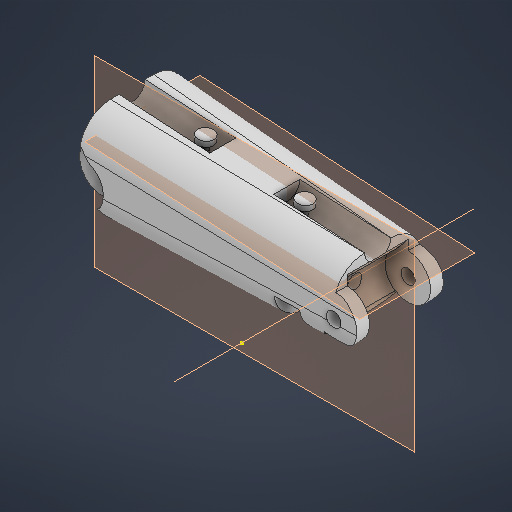
# Autodesk Inventor part: falange1_inidice_V13
Saved by Autodesk Inventor 2026.1 (Build 301233020, 233B)
## iProperties
Created: 2026-01-14
Part Number: falange1_inidice_V13
Material: Generic
Document SubType Name: Modeling
Designer: user
Density: 1 g/cm^3
Appearance: Default
Author: user
Autodesk Inventor part; units mm, degrees
ref_plane "YZ Plane" through (0, 0, 0) normal (1, 0, 0) x (0, 1, 0)
sketch "Sketch1" plane through (0, 0, 0) normal (0, 0, 1) x (1, 0, 0)
  line L0 (5.267598, -7.522909) -> (48.732402, -7.522909)
  circle A0 centre (54, 0) radius 1.575
  arc A1 (0, 5) -> (2.867882, -4.09576) centre (0, 0) ccw
  line L1 (0, 5) -> (0, 12.477091)
  arc A2 (51.175136, -4.034324) -> (54, 4.925) centre (54, 0) ccw
  line L2 (54, 4.925) -> (54, 9.275)
  line L3 (0, 12.477091) -> (54, 9.275)
  line L4 (2.867882, -4.09576) -> (5.267598, -7.522909)
  line L5 (51.175136, -4.034324) -> (48.732402, -7.522909)
  dimension "d31" = 20
  dimension "d39" = 3.15
  dimension "d46" = 10
  dimension "d57" = 12.47709
  dimension "d131" = 54
  dimension "d132" = 9.85
  dimension "d133" = 4.35
  dimension "d176" = 125
  dimension "d186" = 55
  constraints: 12 end point, 4 point on circle, 3 centre point, 2 coincident, 2 vertical, 1 perpendicular
  measures "d31" distance from line of L0 L1.end
  measures "d39" diameter of A0
  measures "d46" diameter of A1
  measures "d57" distance of L1.end point (0, 0)
  measures "d131" distance of A0.centre point (0, 0)
  measures "d132" diameter of A2
  measures "d133" distance of L2.start L2.end
  measures "d176" angle of L0 L4
  measures "d186" angle of L0 L5
extrude "Extrusion1" add sketch "Sketch1" along normal mid plane 23
sketch "Sketch3" plane through (0, 0, 11.5) normal (0, 0, 1) x (1, 0, 0)
  circle A0 centre (0, 0) radius 1.575
  circle A1 centre (0, 0) radius 5
  dimension "d49" = 3.15
  dimension "d50" = 10
  constraints: 2 centre point, 2 coincident
  measures "d49" diameter of A0
  measures "d50" diameter of A1
sketch "Sketch4" plane through (0, 0, -11.5) normal (0, 0, -1) x (-1, 0, 0)
  circle A0 centre (0, 0) radius 1.5
  circle A1 centre (0, 0) radius 5
  dimension "d51" = 10
  dimension "d52" = 3
  constraints: 2 centre point, 2 coincident
  measures "d51" diameter of A1
  measures "d52" diameter of A0
extrude "Extrusion3" cut sketch "Sketch3" against normal blind 4.945 contours A0 | A1
extrude "Extrusion4" cut sketch "Sketch4" against normal blind 4.945 contours A0 | A1
sketch "Sketch8" plane through (0, 0, 11.5) normal (0, 0, 1) x (1, 0, 0)
  line L0 (46.638548, -7.522909) -> (41.267598, -7.522909)
  line L1 (41.267598, -7.522909) -> (41.267598, -1.697299)
  line L2 (41.267598, -1.697299) -> (46.638548, -1.697299)
  line L3 (46.638548, -1.697299) -> (46.638548, -7.522909)
  point P0 (0, 0)
  point P1 (36.274091, -7.522909)
  point P2 (5.267598, -7.522909)
  dimension "d67" = 5.82561
  dimension "d90" = 5.37095
  dimension "d188" = 36
  constraints: 8 end point, 2 parallel, 1 horizontal, 1 perpendicular
  measures "d67" distance of L2.end L0.start
  measures "d90" distance of L1.end L2.end
  measures "d188" distance of L0.end point (5.268, -7.523)
extrude "Extrusion5" cut sketch "Sketch8" against normal through all
sketch "Sketch11" plane through (41.267598, -7.522909, 11.5) normal (1, 0, 0) x (0, 0, -1)
  circle A0 centre (11.5, 2.912805) radius 1.5
  point P0 (11.5, 7.522909)
  point P1 (11.5, 0)
  dimension "d75" = 2.91281
  dimension "d76" = 3
  constraints: 1 centre point
  measures "d75" distance of point (11.5, 0) A0.centre
  measures "d76" diameter of A0
extrude "Extrusion8" cut sketch "Sketch11" against normal through all
sketch "Sketch14" plane through (0, 12.477091, -11.5) normal (-1, 0, 0) x (0, 0, 1)
  circle A0 centre (11.5, -12.477091) radius 1.5
  line L0 (0, 0) -> (23, 0)
  dimension "d92" = 3
  dimension "d166" = 12.47709
  constraints: 1 centre point, 1 coincident
  measures "d92" diameter of A0
  measures "d166" distance from line of L0 point (11.5, -12.477)
sketch "Sketch15" plane through (0, 0, 0) normal (0, 0, 1) x (1, 0, 0)
  circle A0 centre (0, 0) radius 5
  dimension "d93" = 10
  constraints: 1 centre point, 1 coincident
  measures "d93" diameter of A0
extrude "Extrusion11" cut sketch "Sketch15" along normal mid plane 3.825
extrude "Extrusion12" cut sketch "Sketch3" against normal through all contours A0
sketch "Sketch16" plane through (0, 0, -1.9125) normal (0, 0, 1) x (1, 0, 0)
  point P0 (0, 0)
sketch "Sketch17" plane through (0, 0, 0) normal (0, 0, 1) x (1, 0, 0)
  circle A0 centre (0, 0) radius 1.575
  line L0 (-1.651749, 2.630563) -> (1.45226, 2.745738)
  line L1 (1.45226, 2.745738) -> (3.104008, 0.115175)
  line L2 (3.104008, 0.115175) -> (1.651749, -2.630563)
  line L3 (1.651749, -2.630563) -> (-1.45226, -2.745738)
  line L4 (-1.45226, -2.745738) -> (-3.104008, -0.115175)
  line L5 (-3.104008, -0.115175) -> (-1.651749, 2.630563)
  dimension "d102" = 5.38
  constraints: 12 end point, 1 coincident, 13 other
  measures "d102" distance between parallel lines of L3 L0
extrude "Extrusion13" cut sketch "Sketch17" along normal mid plane 8.085 contours A0 | L0 L1 L2 L3 L4 L5
extrude "Extrusion14" cut sketch "Sketch14" against normal through all
sketch "Sketch18" plane through (0, 0, 0) normal (0, 0, 1) x (1, 0, 0)
  circle A0 centre (54, 0) radius 5.075
  circle A1 centre (54, 0) radius 1.575 projected
  point P0 (0, 0)
  dimension "d103" = 10.15
  constraints: 1 centre point
  measures "d103" diameter of A0
extrude "Extrusion15" cut sketch "Sketch18" along normal mid plane 13.41 contours A0 | A1
ref_plane "Work Plane1" through (0, 12.477091, -11.5) normal (0, 1, 0) x (-1, 0, 0)
sketch "Sketch26" plane through (0, 12.477091, -11.5) normal (-1, 0, 0) x (0, 0, 1)
  line L0 (0, 0) -> (23, 0)
  circle A0 centre (11.5, 0) radius 2.860389
  point P0 (11.5, -12.477091)
  dimension "d146" = 5.72078
  constraints: 1 centre point, 1 midpoint
  measures "d146" diameter of A0
sketch "Sketch28" plane through (54, 4.925, -11.5) normal (1, 0, 0) x (0, 0, -1)
  line L0 (-23, 4.35) -> (0, 4.35)
  circle A0 centre (-11.5, 4.35) radius 2.860389
  point P0 (-11.5, -4.925)
  dimension "d147" = 5.72078
  constraints: 1 centre point, 1 midpoint
  measures "d147" diameter of A0
sketch "Sketch29" plane through (0, 12.477091, 11.5) normal (0.059194, 0.9982465, 0) x (0.9982465, -0.059194, 0)
  line L0 (0, 23) -> (0, 0) projected
  line L1 (0, 11.5) -> (20, 11.5)
  point P0 (0.738569, 11.5)
  dimension "d144" = 20
  constraints: 2 end point, 1 horizontal, 1 midpoint
  measures "d144" distance of L1.start L1.end
sketch "Sketch30" plane through (0, 12.477091, 11.5) normal (0.059194, 0.9982465, 0) x (0.9982465, -0.059194, 0)
  line L0 (54.094855, 0) -> (54.094855, 23)
  line L1 (54.094855, 11.5) -> (34.094855, 11.5)
  point P0 (0.738569, 11.5)
  dimension "d145" = 20
  constraints: 2 end point, 1 horizontal, 1 midpoint
  measures "d145" distance of L1.start L1.end
sweep "Sweep2" cut profiles "Sketch26" path "Sketch29" path curves L1
sweep "Sweep3" cut profiles "Sketch28" path "Sketch30" path curves L1
ref_plane "Work Plane3" through (53.830979, 6.424634, 0) normal (0.059194, 0.9982465, 0) x (0.9982465, -0.059194, 0)
sketch "Sketch31" plane through (53.830979, 6.424634, 0) normal (0.059194, 0.9982465, 0) x (0.9982465, -0.059194, 0)
  line L0 (0.248615, -6.705) -> (0.248615, 6.705)
  line L1 (0.248615, 0) -> (-15.991385, 0)
  circle A0 centre (-15.991385, 0) radius 0.732091
  point P0 (-53.356287, 0)
  dimension "d152" = 16.24
  dimension "d153" = 1.46418
  constraints: 2 end point, 1 centre point, 1 coincident, 1 midpoint
  measures "d152" distance of L1.start L1.end
  measures "d153" diameter of A0
extrude "Extrusion23" add sketch "Sketch31" along normal mid plane 3.3575
sketch "Sketch32" plane through (53.830979, 6.424634, 0) normal (0.059194, 0.9982465, 0) x (0.9982465, -0.059194, 0)
  ellipse E0 centre (-54.094855, 0) end of major axis (-54.094855, 2.860389) minor radius 0.169318 (-54.094855, -2.860389) -> (-54.094855, 2.860389) ccw
  circle A0 centre (-37.854855, 0) radius 0.732091
  point P0 (-53.356287, 0)
  dimension "d157" = 1.46418
  dimension "d187" = 16.24
  constraints: 1 centre point, 1 other
  measures "d157" diameter of A0
  measures "d187" distance of A0.centre point (-54.095, 0)
extrude "Extrusion24" add sketch "Sketch32" along normal mid plane 3.3575
sketch "Sketch33" plane through (16.141874, 10.341221, 0) normal (0.059194, 0.9982465, 0) x (0.9982465, -0.059194, 0)
  circle A0 centre (0, 0) radius 0.732091
  circle A1 centre (0, 0) radius 1.774025
  point P0 (-15.501431, 0)
  dimension "d160" = 3.54805
  constraints: 1 centre point, 1 coincident
  measures "d160" diameter of A1
extrude "Extrusion25" add sketch "Sketch33" along normal up to surface (1.176623 mm away) contours A0 | A1
sketch "Sketch34" plane through (37.967007, 9.047035, 0) normal (0.059194, 0.9982465, 0) x (0.9982465, -0.059194, 0)
  circle A0 centre (0, 0) radius 0.732091
  circle A1 centre (0, 0) radius 1.774025
  point P0 (-37.364901, 0)
  dimension "d163" = 3.54805
  constraints: 1 centre point, 1 coincident
  measures "d163" diameter of A1
extrude "Extrusion26" add sketch "Sketch34" along normal up to surface (1.176623 mm away) contours A0 | A1
chamfer "Chamfer1" distance 2 angle 45 1 edges at (54, 5.075, 0)
chamfer "Chamfer2" distance 2 angle 45 2 edges at (0, 5, -9.0275) (0, 5, 9.0275)
sketch "Sketch35" plane through (46.638548, -7.522909, 11.5) normal (-1, 0, 0) x (0, 0, 1)
  line L0 (0, 5.82561) -> (-23, 5.82561)
  line L1 (0, 5.82561) -> (0, 0)
  line L2 (-23, 5.82561) -> (0, 5.82561)
  circle A0 centre (-11.5, 1.996968) radius 1
  point P0 (-11.5, 7.522909)
  dimension "d173" = 2
  constraints: 2 end point, 1 centre point, 1 perpendicular
  measures "d173" diameter of A0
ref_plane "Work Plane4" through (46.638548, -1.697299, 11.5) normal (-0.7071068, 0.7071068, 0) x (0, 0, -1)
sketch "Sketch36" plane through (46.638548, -1.697299, 11.5) normal (-0.7071068, 0.7071068, 0) x (0, 0, -1)
  point P0 (11.5, 31.778262)
sketch3d "3D Sketch1"
sketch "Sketch38" plane through (5.267598, -7.522909, -11.5) normal (0, -1, 0) x (1, 0, 0)
  line L0 (-5.267598, 23) -> (-5.267598, 18.055)
  line L1 (-5.267598, 23) -> (53.657402, 21)
  line L2 (53.657402, 21) -> (53.657402, 11.5)
  line L3 (53.657402, 18.205) -> (53.657402, 23)
  line L4 (-42.701645, 11.5) -> (69.717244, 11.5)
  line L5 (-3.615849, 13.4125) -> (-3.615849, 15.5425)
  line L6 (-5.267598, 0) -> (53.657402, 2)
  line L7 (53.657402, 2) -> (53.657402, 11.5)
  line L8 (-5.267598, 23) -> (-26.641804, 23)
  line L9 (-26.641804, 23) -> (-26.641804, 11.5)
  line L10 (-5.267598, 0) -> (-26.641804, 0)
  line L11 (-26.641804, 0) -> (-26.641804, 11.5)
  point P0 (-5.267598, 11.5)
  dimension "d179" = 9.5
  dimension "d189" = 0
  constraints: 16 end point, 3 symmetric about line, 2 perpendicular, 2 point on line, 1 collinear, 1 horizontal
  measures "d179" distance of L1.end L2.end
  measures "d189" distance from line of L3.start L2
extrude "Extrusion27" cut sketch "Sketch38" against normal through all keep common part
fillet "Fillet1" radius 6.7625 2 edges at (27, 10.876, 10.5836) (27, 10.876, -10.5836)
fillet "Fillet2" radius 6.7625 4 edges at (23.2676, -7.5229, 10.7103) (23.2676, -7.5229, -10.7103) (47.6855, -7.5229, 9.8815) (47.6855, -7.5229, -9.8815)
extrude "Extrusion28" cut sketch "Sketch35" against normal blind 10
equation "\"d39\" = diametroDentroUnion + tolerancia"
equation "\"d46\" = diametroFueraUnion"
equation "\"d132\" = diametroFueraUnion - tolerancia"
equation "\"d49\" = diametroDentroUnion + tolerancia"
equation "\"d50\" = diametroFueraUnion"
equation "\"d51\" = diametroFueraUnion"
equation "\"d52\" = diametroDentroUnion"
equation "\"d93\" = diametroFueraUnion"
equation "\"d103\" = diametroFueraUnion + tolerancia"
equation "\"diametroDentroUnion\" = 3"
equation "\"diametroFueraUnion\" = 10"
equation "\"tolerancia\" = 0.15"
body "Solid1"
